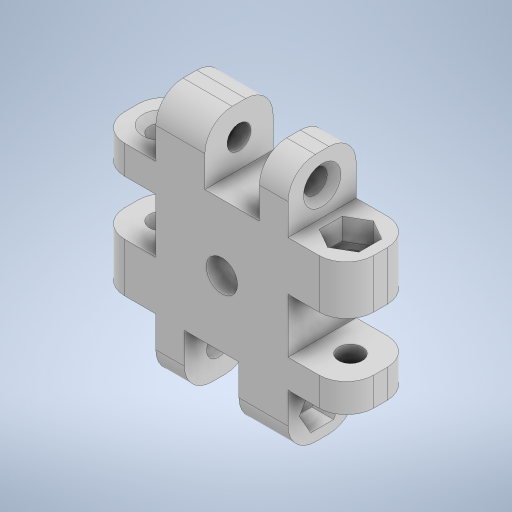
# Autodesk Inventor part: GripperMotorHinges
Saved by Autodesk Inventor 2023 (Build 270158000, 158)
## iProperties
Created: 2023-06-03
Part Number: GripperMotorHinges
Material: Ogólny
Document SubType Name: Modeling
Designer: Kamil
Density: 1 g/cm^3
Appearance: Domyślna
Author: Kamil
Autodesk Inventor part; units mm, degrees
ref_plane "YZ Plane" through (0, 0, 0) normal (1, 0, 0) x (0, 1, 0)
ref_plane "XZ Plane" through (0, 0, 0) normal (0, 1, 0) x (-1, 0, 0)
ref_plane "XY Plane" through (0, 0, 0) normal (0, 0, 1) x (1, 0, 0)
sketch "Szkic1" plane through (0, 0, 0) normal (0, 0, 1) x (1, 0, 0)
  line L0 (0, -7.56) -> (0, 0)
  line L1 (0, 19.4) -> (0, 26.96)
  line L2 (-4.2, 4.2) -> (-11.76, 4.2)
  line L3 (-11.76, 15.2) -> (-4.2, 15.2)
  line L4 (15.2, 15.2) -> (22.76, 15.2)
  line L5 (15.2, 4.2) -> (22.76, 4.2)
  line L6 (-4.2, 26.96) -> (-4.2, 19.4)
  line L7 (-4.2, 19.4) -> (-11.76, 19.4)
  line L8 (-4.2, 15.2) -> (-4.2, 4.2)
  line L9 (-4.2, 0) -> (-4.2, -7.56)
  line L10 (-11.76, 0) -> (-4.2, 0)
  line L11 (15.2, -7.56) -> (11, -7.56)
  line L12 (0, -7.56) -> (-4.2, -7.56)
  line L13 (0, 0) -> (11, 0)
  line L14 (15.2, 0) -> (22.76, 0)
  line L15 (11, 26.96) -> (11, 19.4)
  line L16 (11, 0) -> (11, -7.56)
  line L17 (15.2, -7.56) -> (15.2, 0)
  line L18 (15.2, 4.2) -> (15.2, 15.2)
  line L19 (15.2, 19.4) -> (15.2, 26.96)
  line L20 (22.76, 19.4) -> (15.2, 19.4)
  line L21 (11, 19.4) -> (0, 19.4)
  line L22 (22.76, 19.4) -> (22.76, 15.2)
  line L23 (22.76, 4.2) -> (22.76, 0)
  line L24 (-4.2, 26.96) -> (0, 26.96)
  line L25 (11, 26.96) -> (15.2, 26.96)
  line L26 (-11.76, 0) -> (-11.76, 4.2)
  line L27 (-11.76, 15.2) -> (-11.76, 19.4)
  circle A0 centre (5.5, 9.7) radius 2.3
  dimension "d0" = 4.6
  constraints: 56 end point, 8 parallel, 8 perpendicular, 2 horizontal, 1 centre point, 1 coincident
  measures "d0" diameter of A0
extrude "Wyciągnięcie proste1" add sketch "Szkic1" along normal blind 10
sketch "Szkic2" plane through (-11.76, 19.4, 0) normal (0, 1, 0) x (1, 0, 0)
  line L0 (7.56, 0) -> (0, 0) projected
  line L1 (0, 0) -> (0, -10) projected
  line L2 (7.56, -10) -> (0, -10) projected
  line L3 (7.56, 0) -> (7.56, -10) projected
  line L4 (34.52, 0) -> (26.96, 0) projected
  line L5 (26.96, 0) -> (26.96, -10) projected
  line L6 (34.52, -10) -> (26.96, -10) projected
  line L7 (34.52, 0) -> (34.52, -10) projected
  line L8 (0, 0) -> (0, -10) projected
  line L9 (0, -5) -> (3.4, -5)
  line L10 (34.52, 0) -> (34.52, -10) projected
  line L11 (34.52, -5) -> (31.12, -5)
  circle A0 centre (3.4, -5) radius 1.75
  circle A1 centre (31.12, -5) radius 1.75
  point P0 (11.76, 0)
  dimension "d3" = 3.4
  dimension "d4" = 3.4
  dimension "d5" = 3.5
  dimension "d6" = 3.5
  constraints: 4 end point, 2 centre point, 2 coincident, 2 horizontal, 2 midpoint
  measures "d3" distance of L9.start L9.end
  measures "d4" distance of L11.start L11.end
  measures "d5" diameter of A0
  measures "d6" diameter of A1
extrude "Wyciągnięcie proste2" cut sketch "Szkic2" against normal through all contours A0 | A1
sketch "Szkic3" plane through (-4.2, -7.56, 0) normal (-1, 0, 0) x (0, 0, 1)
  line L0 (0, 7.56) -> (0, 0) projected
  line L1 (0, 0) -> (10, 0) projected
  line L2 (10, 7.56) -> (10, 0) projected
  line L3 (0, 7.56) -> (10, 7.56) projected
  line L4 (0, 34.52) -> (0, 26.96) projected
  line L5 (0, 26.96) -> (10, 26.96) projected
  line L6 (10, 34.52) -> (10, 26.96) projected
  line L7 (0, 34.52) -> (10, 34.52) projected
  line L8 (5, 0) -> (5, 3.4)
  line L9 (0, 34.52) -> (10, 34.52) projected
  line L10 (5, 34.52) -> (5, 31.12)
  circle A0 centre (5, 3.4) radius 1.75
  circle A1 centre (5, 31.12) radius 1.75
  point P0 (0, 7.56)
  dimension "d9" = 3.4
  dimension "d10" = 3.4
  dimension "d11" = 3.5
  dimension "d12" = 3.5
  constraints: 4 end point, 2 centre point, 2 coincident, 2 midpoint, 2 vertical
  measures "d9" distance of L8.start L8.end
  measures "d10" distance of L10.start L10.end
  measures "d11" diameter of A0
  measures "d12" diameter of A1
extrude "Wyciągnięcie proste3" cut sketch "Szkic3" against normal through all contours A0 | A1
sketch "Szkic4" plane through (0, 0, 10) normal (0, 0, 1) x (1, 0, 0)
  line L0 (-4.2, 0) -> (-4.2, -7.56) projected
  line L1 (-4.2, -7.56) -> (0, -7.56) projected
  line L2 (0, -7.56) -> (0, 0) projected
  line L3 (0, 0) -> (11, 0) projected
  line L4 (11, 0) -> (11, -7.56) projected
  line L5 (11, -7.56) -> (15.2, -7.56) projected
  line L6 (15.2, -7.56) -> (15.2, 0) projected
  line L7 (15.2, 0) -> (22.76, 0) projected
  line L8 (22.76, 0) -> (22.76, 4.2) projected
  line L9 (22.76, 4.2) -> (15.2, 4.2) projected
  line L10 (15.2, 4.2) -> (15.2, 15.2) projected
  line L11 (15.2, 15.2) -> (22.76, 15.2) projected
  line L12 (22.76, 15.2) -> (22.76, 19.4) projected
  line L13 (22.76, 19.4) -> (15.2, 19.4) projected
  line L14 (15.2, 19.4) -> (15.2, 26.96) projected
  line L15 (15.2, 26.96) -> (11, 26.96) projected
  line L16 (11, 26.96) -> (11, 19.4) projected
  line L17 (11, 19.4) -> (0, 19.4) projected
  line L18 (0, 19.4) -> (0, 26.96) projected
  line L19 (0, 26.96) -> (-4.2, 26.96) projected
  line L20 (-4.2, 26.96) -> (-4.2, 19.4) projected
  line L21 (-4.2, 19.4) -> (-11.76, 19.4) projected
  line L22 (-11.76, 19.4) -> (-11.76, 15.2) projected
  line L23 (-11.76, 15.2) -> (-4.2, 15.2) projected
  line L24 (-4.2, 15.2) -> (-4.2, 4.2) projected
  line L25 (-4.2, 4.2) -> (-11.76, 4.2) projected
  line L26 (-11.76, 4.2) -> (-11.76, 0) projected
  line L27 (-11.76, 0) -> (-4.2, 0) projected
  circle A0 centre (5.5, 9.7) radius 2.3 projected
  line L28 (0, 19.4) -> (0, 26.96) projected
  line L29 (11, 19.4) -> (0, 19.4) projected
  line L30 (0, 26.96) -> (3, 26.96)
  line L31 (3, 26.96) -> (3, 19.4)
  line L32 (3, 19.4) -> (0, 19.4)
  line L33 (0, 19.4) -> (0, 26.96)
  line L34 (11, 0) -> (8, 0)
  line L35 (8, 0) -> (8, -7.56)
  line L36 (8, -7.56) -> (11, -7.56)
  line L37 (11, -7.56) -> (11, 0)
  line L38 (15.2, 15.2) -> (22.76, 15.2)
  line L39 (22.76, 15.2) -> (22.76, 12.2)
  line L40 (22.76, 12.2) -> (15.2, 12.2)
  line L41 (15.2, 12.2) -> (15.2, 15.2)
  line L42 (-4.2, 4.2) -> (-11.76, 4.2)
  line L43 (-11.76, 4.2) -> (-11.76, 7.2)
  line L44 (-11.76, 7.2) -> (-4.2, 7.2)
  line L45 (-4.2, 7.2) -> (-4.2, 4.2)
  dimension "d15" = 3
  dimension "d16" = 3
  dimension "d17" = 3
  dimension "d18" = 3
  constraints: 32 end point, 8 parallel, 4 horizontal, 4 perpendicular, 1 point on line
  measures "d15" distance of L31.end L32.end
  measures "d16" distance of L36.end L35.end
  measures "d17" distance of L38.end L39.end
  measures "d18" distance of L42.end L43.end
extrude "Wyciągnięcie proste4" add sketch "Szkic4" against normal up to surface (10 mm away) contours L43 L44 L24 L25 | L3 L4 L36 L35 | L30 L31 L17 L18 | L10 L11 L39 L40
sketch "Szkic5" plane through (-4.2, 19.4, 0) normal (-1, 0, 0) x (0, 0, 1)
  circle A0 centre (5, 4.16) radius 1.75 projected
  line L0 (0, 7.56) -> (0, 0) projected
  line L1 (0, 0) -> (10, 0) projected
  line L2 (10, 7.56) -> (10, 0) projected
  line L3 (0, 7.56) -> (10, 7.56) projected
  circle A1 centre (5, 4.16) radius 2.9
  circle A2 centre (5, 4.16) radius 1.75 projected
  line L4 (6.6743, 7.06) -> (8.3486, 4.16)
  line L5 (8.3486, 4.16) -> (6.6743, 1.26)
  line L6 (6.6743, 1.26) -> (3.3257, 1.26)
  line L7 (3.3257, 1.26) -> (1.6514, 4.16)
  line L8 (1.6514, 4.16) -> (3.3257, 7.06)
  line L9 (3.3257, 7.06) -> (6.6743, 7.06)
  point P0 (0, -19.4)
  point P1 (5, 7.06)
  dimension "d21" = 5.8
  constraints: 12 end point, 2 coincident, 1 midpoint, 1 vertical alignment, 15 other
extrude "Wyciągnięcie proste5" cut sketch "Szkic5" against normal blind 3.2 contours A0 | A1 | A1 L4 L5 | A1 L9 L4 | L5 L6 A1 | A1 L8 L9 | L6 L7 A1 | A1 L7 L8
sketch "Szkic6" plane through (-1, 19.4, 0) normal (-1, 0, 0) x (0, 0, 1)
  circle A0 centre (5, 4.16) radius 1.75 projected
  point P0 (0, -19.4)
extrude "Wyciągnięcie proste6" cut sketch "Szkic6" against normal through all
pattern_circular "Szyk kołowy1" count 4 over 360 about axis through (5.5, 9.7, 0) along (0, 0, 1) of "Wyciągnięcie proste6", "Wyciągnięcie proste5"
sketch "Szkic7" plane through (-4.2, 26.96, 10) normal (0, 1, 0) x (1, 0, 0)
  line L0 (0, 10) -> (7.2, 10) projected
  line L1 (0, 10) -> (0, 0) projected
  line L2 (7.2, 0) -> (0, 0) projected
  line L3 (7.2, 0) -> (7.2, 10) projected
  line L4 (19.4, 10) -> (15.2, 10) projected
  line L5 (15.2, 10) -> (15.2, 0) projected
  line L6 (19.4, 0) -> (15.2, 0) projected
  line L7 (19.4, 10) -> (19.4, 0) projected
  point P0 (4.2, 10)
extrude "Wyciągnięcie proste7" add sketch "Szkic7" along normal blind 1
pattern_circular "Szyk kołowy2" count 4 over 360 about axis through (5.5, 9.7, 0) along (0, 0, 1) of "Wyciągnięcie proste7"
chamfer "Faza1" distance 1 angle 45 4 edges at (-10.11, 19.4, 5) (-4.2, -4.16, 3.25) (17.61, 0, 5) (15.2, 23.56, 3.25)
fillet "Zaokrąglenie1" radius 4 4 edges at (-12.76, 3.6, 0) (11.6, -8.56, 0) (23.76, 15.8, 0) (-0.6, 27.96, 0)
fillet "Zaokrąglenie2" radius 4 12 edges at (11.6, -8.56, 10) (-2.1, -8.56, 10) (-2.1, -8.56, 0) (23.76, 2.1, 10) (23.76, 2.1, 0) (23.76, 15.8, 10) (13.1, 27.96, 10) (13.1, 27.96, 0) (-0.6, 27.96, 10) (-12.76, 17.3, 10) (-12.76, 3.6, 10) (-12.76, 17.3, 0)
